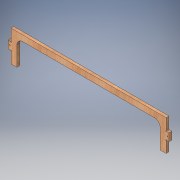
# Autodesk Inventor part: bottom
Saved by Autodesk Inventor 2016 (Build 200138000, 138)
## iProperties
Created: 2017-03-13
Part Number: bottom
Material: Wood (Birch)
Document SubType Name: Modeling
Designer: jwillauer
Density: 0.55 g/cm^3
Appearance: Birch - Natural Polished
Author: jwillauer
Autodesk Inventor part; units mm, degrees
ref_plane "YZ Plane" through (0, 0, 0) normal (1, 0, 0) x (0, 1, 0)
ref_plane "XZ Plane" through (0, 0, 0) normal (0, 1, 0) x (-1, 0, 0)
ref_plane "XY Plane" through (0, 0, 0) normal (0, 0, 1) x (1, 0, 0)
sketch "Sketch1" plane through (0, 0, 0) normal (0, 0, 1) x (1, 0, 0)
  line L0 (-48.4923, 85.7611) -> (-48.4923, 34.9611)
  line L1 (-48.4923, 34.9611) -> (-29.6963, 34.9611)
  line L2 (-29.6963, 34.9611) -> (-29.6963, -41.2389)
  line L3 (-29.6963, -41.2389) -> (986.3037, -41.2389)
  line L4 (986.3037, -41.2389) -> (986.3037, 34.9611)
  line L5 (986.3037, 34.9611) -> (1005.0997, 34.9611)
  line L6 (1005.0997, 34.9611) -> (1005.0997, 85.7611)
  line L7 (1005.0997, 85.7611) -> (986.3037, 85.7611)
  line L8 (986.3037, 85.7611) -> (986.3037, 161.9611)
  line L9 (986.3037, 161.9611) -> (-29.6963, 161.9611)
  line L10 (-48.4923, 85.7611) -> (-29.6963, 85.7611)
  line L11 (-29.6963, 85.7611) -> (-29.6963, 161.9611)
  point P0 (0, 0)
  dimension "d0" = 50.8
  dimension "d1" = 18.796
  dimension "d2" = 76.2
  dimension "d3" = 1016
  dimension "d4" = 76.2
  dimension "d5" = 18.796
  dimension "d6" = 50.8
  dimension "d7" = 76.2
  dimension "d8" = 18.796
  constraints: 24 end point, 8 perpendicular, 2 horizontal, 2 vertical
  measures "d0" distance of L0.start L0.end
  measures "d1" distance of L0.end L1.end
  measures "d2" distance of L1.end L2.end
  measures "d3" distance of L2.end L3.end
  measures "d4" distance of L3.end L4.end
  measures "d5" distance of L4.end L5.end
  measures "d6" distance of L5.end L6.end
  measures "d7" distance of L7.end L8.end
  measures "d8" distance of L6.end L7.end
extrude "Extrusion1" add sketch "Sketch1" along normal blind 18.796
sketch "Sketch2" plane through (0, 0, 18.796) normal (0, 0, 1) x (1, 0, 0)
  line L0 (-29.6963, 85.7611) -> (-48.4923, 85.7611) projected
  line L1 (-48.4923, 34.9611) -> (-29.6963, 34.9611) projected
  line L2 (1005.0997, 34.9611) -> (1005.0997, 85.7611) projected
  line L3 (-48.4923, 85.7611) -> (-48.4923, 34.9611) projected
  point P0 (0, 0)
  point P1 (-39.0943, 60.5407)
  point P2 (986.9445, 85.7611)
  point P3 (986.9445, 34.9611)
  point P4 (995.7017, 60.5407)
  dimension "d11" = 9.398
  dimension "d12" = 9.398
  measures "d11" distance from line of L2 point (995.702, 60.541)
  measures "d12" distance from line of L3 point (-39.094, 60.541)
hole "Hole1" at (-29.6963, 85.7611, 18.796) at (-29.6963, 34.9611, 18.796) at (-39.0943, 60.5407, 18.796) at (986.9445, 85.7611, 18.796) at (986.9445, 34.9611, 18.796) at (995.7017, 60.5407, 18.796) direction (0, 0, -1) diameter 6.35 end through all
sketch "Sketch3" plane through (0, 0, 18.796) normal (0, 0, 1) x (1, 0, 0)
  line L0 (-29.6963, -41.2389) -> (986.3037, -41.2389) projected
  line L1 (8.4037, -41.2389) -> (948.2037, -41.2389)
  line L2 (948.2037, -41.2389) -> (948.2037, 85.7611)
  line L3 (910.1037, 123.8611) -> (46.5037, 123.8611)
  line L4 (8.4037, 85.7611) -> (8.4037, -41.2389)
  line L5 (-29.6963, 31.7861) -> (-29.6963, -41.2389) projected
  line L6 (986.3037, -41.2389) -> (986.3037, 31.8515) projected
  arc A0 (11.5787, 123.8611) -> (8.4037, 120.6861) centre (11.5787, 120.6861) ccw
  arc A1 (46.5037, 123.8611) -> (8.4037, 85.7611) centre (46.5037, 85.7611) ccw
  arc A2 (948.2037, 85.7611) -> (910.1037, 123.8611) centre (910.1037, 85.7611) ccw
  point P0 (0, 0)
  point P1 (948.2037, 123.8611)
  point P2 (8.4037, 123.8611)
  dimension "d20" = 38.1
  dimension "d21" = 38.1
  dimension "d22" = 939.8
  dimension "d23" = 165.1
  dimension "d24" = 3.175
  dimension "d25" = 38.1
  constraints: 8 end point, 7 point on line, 6 point on circle, 6 tangent, 3 centre point, 2 parallel, 1 equal radius, 1 horizontal, 1 perpendicular
  measures "d20" distance between parallel lines of L5 L4
  measures "d21" distance between parallel lines of L6 L2
  measures "d22" distance of point (948.204, 123.861) point (8.404, 123.861)
  measures "d23" distance between parallel lines of L0 L3
  measures "d24" radius of A0
  measures "d25" radius of A1
extrude "Extrusion2" cut sketch "Sketch3" against normal blind 25.4
body "Solid1"
